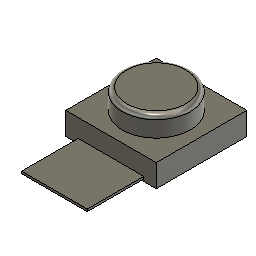
verdure-buddy (Autodesk Fusion 360 archive; units mm, degrees)
design "官方摄像头"
Autodesk Fusion 360 part; units mm, degrees
sketch "草图1" plane through (0, 0, 0) normal (0, 1, 0) x (1, 0, 0)
  line L0 (4, -4) -> (-4, -4)
  line L1 (-4, -4) -> (-4, 4)
  line L2 (-4, 4) -> (4, 4)
  line L3 (4, 4) -> (4, -4)
  line L4 (4, -4) -> (-4, 4) construction
  line L5 (-4, -4) -> (4, 4) construction
  circle A0 centre (0, 0) radius 3
  line L6 (-2.9, -4) -> (2.9, -4)
  line L7 (2.9, -4) -> (2.9, -9)
  line L8 (2.9, -9) -> (-2.9, -9)
  line L9 (-2.9, -9) -> (-2.9, -4)
  dimension "d1" = 8
  dimension "d2" = 8
  dimension "d3" = 6
  dimension "d4" = 5.8
  dimension "d5" = 5
  dimension "d6" = 1.1
  constraint horizontal L0
  constraint perpendicular L0 L1
  constraint parallel L0 L2
  constraint parallel L1 L3
  constraint coincident L4 A0.centre
  constraint coincident L5 A0.centre
  constraint coincident A0.centre origin
  constraint horizontal L6
  constraint vertical L7
  constraint horizontal L8
  constraint vertical L9
  constraint coincident L0 L6.start
  measures "d1" distance of L1.end L2.end
  measures "d2" distance of L0.end L1.end
  measures "d3" diameter of A0
  measures "d4" distance of L6.start L6.end
  measures "d5" distance of L6.start L8.end
  measures "d6" distance of L0.end L6.start
extrude "拉伸1" add sketch "草图1" against normal blind 2 contours L0 L1 L2 L3 L6 | A0
extrude "拉伸2" add sketch "草图1" along normal blind 1.8 contours A0
extrude "拉伸3" add sketch "草图1" against normal blind 1.8 contours L0 L6 L7 L8 L9
extrude "拉伸4" cut sketch "草图1" against normal blind 1.6 contours L0 L6 L7 L8 L9
fillet "圆角1" radius 0.4 1 edges at (-2.797, 1.8, 1.0848)

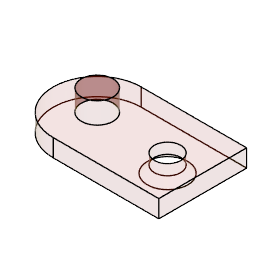
design "导光柱"
Autodesk Fusion 360 part; units mm, degrees
sketch "草图1" plane through (0, 0, 0) normal (0, 1, 0) x (1, 0, 0)
  line L0 (4.25, -2.5) -> (-4.25, -2.5)
  line L1 (-4.25, -2.5) -> (-4.25, 2.5)
  line L2 (-4.25, 2.5) -> (4.25, 2.5)
  line L3 (4.25, 2.5) -> (4.25, -2.5)
  line L4 (4.25, -2.5) -> (-4.25, 2.5) construction
  line L5 (-4.25, -2.5) -> (4.25, 2.5) construction
  dimension "d1" = 8.5
  dimension "d2" = 5
  constraint horizontal L0
  constraint perpendicular L0 L1
  constraint parallel L0 L2
  constraint parallel L1 L3
  constraint coincident L4 origin
  constraint coincident L5 origin
  measures "d1" distance of L1.end L2.end
  measures "d2" distance of L0.end L1.end
extrude "拉伸1" add sketch "草图1" along normal blind 1
sketch "草图2" plane through (0, 1, 0) normal (0, 1, 0) x (-1, 0, 0)
  line L0 (-4.25, -2.5) -> (4.25, -2.5)
  line L1 (4.25, -2.5) -> (4.25, 2.5)
  line L2 (4.25, 2.5) -> (-4.25, 2.5)
  line L3 (-4.25, 2.5) -> (-4.25, -2.5)
  circle A0 centre (-2.25, 0) radius 0.75
  circle A1 centre (1.75, 0) radius 0.9
  dimension "d5" = 1.5
  dimension "d6" = 2
  dimension "d7" = 1.8
  dimension "d8" = 4
  measures "d5" diameter of A0
  measures "d6" distance of L3 A0.centre
  measures "d7" diameter of A1
  measures "d8" distance of A0.centre A1.centre
extrude "拉伸2" add sketch "草图2" along normal blind 1.2 contours A1
extrude "拉伸3" cut sketch "草图2" against normal blind 3.5 contours A0
chamfer "倒角1" distance 0.4 angle 45 1 edges at (2.9492, 0, -0.2712)
fillet "圆角1" radius 2.5 2 edges at (-4.25, 0.5, 2.5) (-4.25, 0.5, -2.5)
